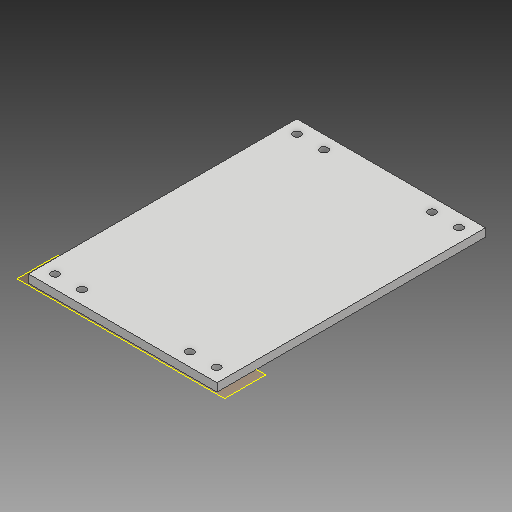
# Autodesk Inventor part: 20_Projector_Sony_Moun_2
Saved by Autodesk Inventor 2019 (Build 230136000, 136)
## iProperties
Created: 2018-08-23
Part Number: 20_Projector_Sony_Moun_2
Material: Generisch
Document SubType Name: Modeling
Designer: diederichbenedict
Density: 1 g/cm^3
Appearance: Vorgabe
Author: diederichbenedict
Autodesk Inventor part; units mm, degrees
ref_plane "YZ Plane" through (0, 0, 0) normal (1, 0, 0) x (0, 1, 0)
ref_plane "XZ Plane" through (0, 0, 0) normal (0, 1, 0) x (-1, 0, 0)
ref_plane "XY Plane" through (0, 0, 0) normal (0, 0, 1) x (1, 0, 0)
ref_plane "Arbeitsebene1" through (0, 0, 0) normal (0, 0, 1) x (1, 0, 0)
sketch "Skizze1" plane through (0, 0, 0) normal (0, 0, 1) x (1, 0, 0)
  circle A0 centre (-20, -44.9) radius 1.75 projected
  circle A1 centre (30, -44.9) radius 1.75 projected
  circle A2 centre (20, -44.9) radius 1.75 projected
  circle A3 centre (-30, -44.9) radius 1.75 projected
  line L0 (-35, -49.8) -> (-35, -35.9) projected
  line L1 (35, -49.8) -> (-35, -49.8) projected
  line L2 (35, -35.9) -> (35, -49.8) projected
  line L3 (-35, -35.9) -> (35, -35.9) projected
  arc A4 (-19.0986, 43.4) -> (-20.9014, 43.4) centre (-20, 44.9) ccw projected
  line L4 (19.0986, 43.4) -> (-19.0986, 43.4) projected
  arc A5 (20.9014, 43.4) -> (19.0986, 43.4) centre (20, 44.9) ccw projected
  line L5 (29.0986, 43.4) -> (20.9014, 43.4) projected
  arc A6 (30.9014, 43.4) -> (29.0986, 43.4) centre (30, 44.9) ccw projected
  line L6 (35, 43.4) -> (30.9014, 43.4) projected
  line L7 (35, 49.8) -> (35, 43.4) projected
  line L8 (-35, 49.8) -> (35, 49.8) projected
  line L9 (-35, 43.4) -> (-35, 49.8) projected
  line L10 (-30.9014, 43.4) -> (-35, 43.4) projected
  arc A7 (-29.0986, 43.4) -> (-30.9014, 43.4) centre (-30, 44.9) ccw projected
  line L11 (-20.9014, 43.4) -> (-29.0986, 43.4) projected
  line L12 (35, -49.8) -> (-35, -49.8)
  line L13 (-35, -49.8) -> (-35, 49.8)
  line L14 (-35, 49.8) -> (35, 49.8)
  line L15 (35, 49.8) -> (35, -49.8)
  point P0 (0, 0)
  constraints: 8 end point, 2 parallel, 1 horizontal, 1 perpendicular
extrude "Extrusion1" add sketch "Skizze1" along normal blind 3 contours A0 | A1 | A2 | A3 | L0 L3 L2 L1 | L13 L10 A7 L11 A4 L4 A5 L5 A6 L6 L15 L3 | L9 L8 L7 L6 A6 L5 A5 L4 A4 L11 A7 L10
sketch "Skizze2" plane through (0, 0, 3) normal (0, 0, 1) x (1, 0, 0)
  circle A0 centre (30, -44.9) radius 1.75 projected
  circle A1 centre (20, -44.9) radius 1.75 projected
  circle A2 centre (-20, -44.9) radius 1.75 projected
  circle A3 centre (-30, -44.9) radius 1.75 projected
  arc A4 (30.9014, 43.4) -> (29.0986, 43.4) centre (30, 44.9) ccw projected
  arc A5 (20.9014, 43.4) -> (19.0986, 43.4) centre (20, 44.9) ccw projected
  arc A6 (-19.0986, 43.4) -> (-20.9014, 43.4) centre (-20, 44.9) ccw projected
  arc A7 (-29.0986, 43.4) -> (-30.9014, 43.4) centre (-30, 44.9) ccw projected
  point P0 (0, 0)
  constraints: 2 other
hole "Bohrung1" at (30, 44.9, 3) at (20, 44.9, 3) at (-30, -44.9, 3) at (-20, -44.9, 3) at (20, -44.9, 3) at (30, -44.9, 3) at (-20, 44.9, 3) at (-30, 44.9, 3) direction (0, 0, -1) diameter 2.9 end through all
